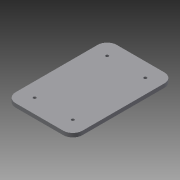
# Autodesk Inventor part: support
Saved by Autodesk Inventor 2013 (Build 170138000, 138)
## iProperties
Created: 2013-06-25
Part Number: support
Material: Generic
Document SubType Name: Modeling
Designer: Piotr
Density: 1 g/cm^3
Mass: 27.7206 g
Surface Area: 159.065 cm^2
Volume: 27.7206 cm^3
Author: Piotr
Autodesk Inventor part; units mm, degrees
ref_plane "YZ Plane" through (0, 0, 0) normal (1, 0, 0) x (0, 1, 0)
ref_plane "XZ Plane" through (0, 0, 0) normal (0, 1, 0) x (-1, 0, 0)
ref_plane "XY Plane" through (0, 0, 0) normal (0, 0, 1) x (1, 0, 0)
sketch "Sketch1" plane through (0, 0, 0) normal (0, 0, 1) x (1, 0, 0)
  line L0 (0, 53.2) -> (0, -53.2) projected
  line L1 (-28, 0) -> (28, 0) projected
  point P0 (0, 0)
  point P1 (20, 38)
  point P2 (-20, 38)
  point P3 (-20, -38)
  point P4 (20, -38)
  dimension "d0" = 76
  dimension "d2" = 40
  constraints: 2 horizontal alignment, 2 symmetric about line, 2 vertical alignment
  measures "d0" distance of point (-20, -38) point (-20, 38)
  measures "d2" distance of point (20, 38) point (-20, 38)
sketch "Sketch2" plane through (0, 0, 0) normal (0, 0, 1) x (1, 0, 0)
  line L0 (-35, 53) -> (35, 53)
  line L1 (35, 53) -> (35, -53)
  line L2 (35, -53) -> (-35, -53)
  line L3 (-35, -53) -> (-35, 53)
  point P0 (0, 0)
  point P1 (-20, 38)
  point P2 (20, 38)
  point P3 (20, -38)
  point P4 (-20, -38)
  dimension "d3" = 15
  dimension "d4" = 15
  dimension "d5" = 15
  dimension "d6" = 15
  constraints: 8 end point, 2 parallel, 1 horizontal, 1 perpendicular
  measures "d3" distance from line of L0 point (20, 38)
  measures "d4" distance from line of point (20, -38) L2
  measures "d5" distance from line of L1 point (20, 38)
  measures "d6" distance from line of L3 point (-20, 38)
extrude "Extrusion1" add sketch "Sketch2" along normal blind 4
hole "Hole1" at (20, 38, 0) at (-20, 38, 0) at (-20, -38, 0) at (20, -38, 0) direction (0, 0, 1) diameter 12 depth 2
hole "Hole2" at (20, 38, 2) direction (0, 0, 1) diameter 3.1 end through all
mirror "Mirror1" about plane through (0, 0, 0) normal (0, 1, 0) of "Hole2"
mirror "Mirror2" about plane through (0, 0, 0) normal (1, 0, 0) of "Hole2", "Mirror1"
fillet "Fillet1" radius 10 4 edges at (35, -53, 2) (-35, -53, 2) (35, 53, 2) (-35, 53, 2)
equation "\"d4\" = d3"
equation "\"d5\" = d3"
equation "\"d6\" = d3"
body "Solid1"
